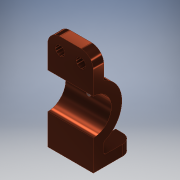
# Autodesk Inventor part: T05
Saved by Autodesk Inventor 2018 (Build 220112000, 112)
## iProperties
Created: 2020-06-25
Part Number: T05
Material: Generic
Document SubType Name: Modeling
Designer: Diego
Density: 1 g/cm^3
Appearance: Copper - Polished
Author: Diego
Autodesk Inventor part; units mm, degrees
ref_plane "YZ Plane" through (0, 0, 0) normal (1, 0, 0) x (0, 1, 0)
ref_plane "XZ Plane" through (0, 0, 0) normal (0, 1, 0) x (-1, 0, 0)
ref_plane "XY Plane" through (0, 0, 0) normal (0, 0, 1) x (1, 0, 0)
sketch "Sketch1" plane through (0, 0, 0) normal (1, 0, 0) x (0, 1, 0)
  line L0 (41, 0) -> (0, 0)
  line L1 (0, 0) -> (0, 32)
  arc A0 (0, 32) -> (0, 70) centre (0, 51) ccw
  line L2 (0, 70) -> (0, 107)
  line L3 (41, 11) -> (11, 11)
  line L4 (11, 11) -> (11, 23.0894)
  arc A1 (11, 23.0894) -> (11, 78.9106) centre (0, 51) ccw
  line L5 (11, 78.9106) -> (11, 107)
  line L6 (11, 107) -> (0, 107)
  line L7 (41, 11) -> (41, 0)
  dimension "d0" = 41
  dimension "d1" = 107
  dimension "d2" = 51
  dimension "d3" = 11
  dimension "d4" = 30
  constraints: 16 end point, 4 perpendicular, 4 point on circle, 3 point on line, 2 centre point, 1 horizontal, 3 other
  measures "d0" distance of L0.start L0.end
  measures "d1" distance of L2.end L0.end
  measures "d2" distance of A0.centre L0.end
  measures "d3" distance between parallel lines of L2 L5
  measures "d4" radius of A1
extrude "Extrusion1" add sketch "Sketch1" along normal mid plane 48
fillet "Fillet1" radius 13 2 edges at (24, 5.5, 107) (-24, 5.5, 107)
fillet "Fillet2" radius 2 3 edges at (0, 11, 78.9106) (0, 11, 23.0894) (0, 11, 11)
sketch "Sketch2" plane through (-11, 11, 107) normal (0, 1, 0) x (1, 0, 0)
  arc A0 (-13, 13) -> (0, 0) centre (0, 13) ccw projected
  circle A1 centre (0, 13) radius 5
  circle A2 centre (22, 13.2869) radius 5
  point P0 (11, 107)
  dimension "d9" = 10
  dimension "d10" = 10
  constraints: 2 centre point, 1 coincident
  measures "d9" diameter of A1
  measures "d10" diameter of A2
extrude "Extrusion2" cut sketch "Sketch2" against normal through all
sketch "Sketch3" plane through (24, 41, 0) normal (0, 0, -1) x (-1, 0, 0)
  line L0 (48, 0) -> (0, 0) projected
  line L1 (24, 0) -> (24, -16) construction
  line L2 (30.5, 0) -> (17.5, 0)
  line L3 (17.5, 0) -> (17.5, -16)
  line L4 (30.5, -16) -> (30.5, 0)
  arc A0 (17.5, -16) -> (30.5, -16) centre (24, -16) ccw
  point P0 (24, -41)
  dimension "d14" = 13
  dimension "d15" = 6.5
  dimension "d16" = 16
  dimension "d17" = 6.5
  constraints: 8 end point, 2 point on circle, 1 centre point, 1 coincident, 1 horizontal, 1 midpoint, 1 parallel, 1 perpendicular, 1 point on line, 1 vertical
  measures "d14" distance between parallel lines of L4 L3
  measures "d15" distance from line of L1 L2.end
  measures "d16" distance of A0.centre L1.start
  measures "d17" radius of A0
extrude "Extrusion3" cut sketch "Sketch3" against normal blind 11
fillet "Fillet3" radius 10 2 edges at (24, 41, 5.5) (-24, 41, 5.5)
sketch "Sketch4" plane through (-24, 0, 0) normal (0, -1, 0) x (1, 0, 0)
  line L0 (48, 70) -> (48, 32) projected
  line L1 (48, 51) -> (0, 51)
  line L2 (0, 78.4129) -> (0, 23.5871) projected
  circle A0 centre (24, 51) radius 2.5
  point P0 (24, 0)
  dimension "d21" = 5
  constraints: 3 midpoint, 2 end point, 1 centre point
  measures "d21" diameter of A0
extrude "Extrusion4" cut sketch "Sketch4" against normal through all
thread "Thread1" size "M5x0.8" class "6H" standard "ISO Metric profile" full length
body "Solid1"
